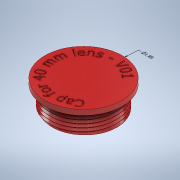
# Autodesk Inventor part: CapForSvBonyPlosse-40mm
Saved by Autodesk Inventor 2021.1 (Build 251245010, 245A)
## iProperties
Created: 2020-10-08
Part Number: CapForSvBonyPlosse-40mm
Material: PC/ABS Plastic
Document SubType Name: Modeling
Designer: robst
Density: 0.357273 g/cm^3
Appearance: Red
Author: robst
Autodesk Inventor part; units mm, degrees
ref_plane "YZ Plane" through (0, 0, 0) normal (1, 0, 0) x (0, 1, 0)
ref_plane "XZ Plane" through (0, 0, 0) normal (0, 1, 0) x (-1, 0, 0)
ref_plane "XY Plane" through (0, 0, 0) normal (0, 0, 1) x (1, 0, 0)
sketch "Sketch7" plane through (0, 0, 0) normal (0, 0, 1) x (1, 0, 0)
  line L0 (0, 0) -> (20.3518, 0)
  line L1 (20.3518, 0) -> (20.3517, 12.7)
  line L2 (20.3517, 12.7) -> (23.5267, 12.7)
  line L3 (23.5267, 12.7) -> (23.5267, 15.875)
  line L4 (23.5267, 15.875) -> (0, 15.875)
  line L5 (20.3518, 0) -> (17.1768, 0)
  line L6 (17.1768, 0) -> (17.1768, 12.7)
  line L7 (17.1768, 12.7) -> (0, 12.7)
  line L8 (0, 15.875) -> (0, 12.7)
  line L9 (0, -10.4241) -> (0, 20.2582) projected
  dimension "d71" = 3.175
  dimension "d72" = 12.7
  dimension "d73" = 20.3517
  dimension "d77" = 3.175
  dimension "d78" = 3.175
  constraints: 18 end point, 5 perpendicular, 2 vertical, 1 horizontal, 1 point on line
  measures "d71" distance between parallel lines of L4 L2
  measures "d72" distance from line of L2 L0.start
  measures "d73" distance of L0.start L0.end
  measures "d77" distance of L2.end L1.end
  measures "d78" distance between parallel lines of L1 L6
revolve "Revolution3" add sketch "Sketch7" angle 360 about axis through (0, -10, 0) along (0, 1, 0) contours L6 L7 L8 L4 L3 L2 L1 L0
sketch "Sketch10" plane through (0, 0, 0) normal (0, 0, 1) x (1, 0, 0)
  line L0 (20.3517, 12.7) -> (20.3517, 0) projected
  line L1 (20.3517, -2.1167) -> (20.3517, -4.1301)
  line L2 (20.3517, -4.1301) -> (18.9433, -3.317)
  line L3 (18.9433, -2.9298) -> (20.3517, -2.1167)
  line L4 (-20.3518, 0) -> (20.3517, 0) projected
  arc A0 (18.9433, -2.9298) -> (18.9433, -3.317) centre (19.0551, -3.1234) ccw
  line L5 (0, -7.921) -> (0, 19.841) projected
  point P0 (0, 0)
  dimension "d100" = 60
  dimension "d101" = 2.1167
  dimension "d102" = 0.2235
  dimension "d103" = 18.8316
  constraints: 6 end point, 2 point on circle, 2 tangent, 1 centre point, 1 collinear, 1 equal length, 1 vertical
  measures "d100" angle of L3 L2
  measures "d101" distance from line of L1.start L4
  measures "d102" radius of A0
  measures "d103" distance edge to line of A0 L5
coil "Coil6" sketch "Sketch10" operation cut axis through (0, -10, 0) along (0, 1, 0) pitch 2.1167 turns 8 hand right
sketch "Sketch11" plane through (0, 15.875, 0) normal (0, 1, 0) x (1, 0, 0)
  circle A0 centre (0, 0) radius 19.05 construction
  spline S0 degree 2 poles (10.2758, -12.8128) (10.6535, -12.4944) (11.5074, -12.2107) (11.9552, -12.2693) knots 0 0 0 1 2 2 2
  spline S1 degree 2 poles (11.9552, -12.2693) (12.4004, -12.3248) (13.2921, -12.8653) (13.7061, -13.3563) knots 0 0 0 1 2 2 2
  spline S2 degree 2 poles (13.7061, -13.3563) (14.1173, -13.8442) (14.4789, -14.7777) (14.4684, -15.2443) knots 0 0 0 1 2 2 2
  spline S3 degree 2 poles (14.4684, -15.2443) (14.4557, -15.7018) (14.0507, -16.5116) (13.6573, -16.8433) knots 0 0 0 1 2 2 2
  spline S4 degree 2 poles (13.6573, -16.8433) (13.4621, -17.0078) (13.0713, -17.2404) (12.8893, -17.3184) knots 0 0 0 1 2 2 2
  spline S5 degree 2 poles (12.8893, -17.3184) (12.729, -17.3836) (12.3695, -17.4873) (12.1821, -17.5269) knots 0 0 0 1 2 2 2
  line L0 (12.1821, -17.5269) -> (11.6568, -16.9037)
  line L1 (11.6568, -16.9037) -> (11.6977, -16.8692)
  spline S6 degree 2 poles (11.6977, -16.8692) (11.82, -16.8737) (12.1826, -16.8696) (12.4085, -16.8245) knots 0 0 0 1 2 2 2
  spline S7 degree 2 poles (12.4085, -16.8245) (12.6254, -16.7817) (13.0623, -16.591) (13.289, -16.4) knots 0 0 0 1 2 2 2
  spline S8 degree 2 poles (13.289, -16.4) (13.5376, -16.1904) (13.809, -15.6117) (13.8113, -15.2759) knots 0 0 0 1 2 2 2
  spline S9 degree 2 poles (13.8113, -15.2759) (13.8078, -14.9396) (13.4836, -14.1846) (13.1678, -13.81) knots 0 0 0 1 2 2 2
  spline S10 degree 2 poles (13.1678, -13.81) (12.8309, -13.4103) (12.1533, -12.9961) (11.8193, -12.9384) knots 0 0 0 1 2 2 2
  spline S11 degree 2 poles (11.8193, -12.9384) (11.4938, -12.8844) (10.8918, -13.0581) (10.6463, -13.265) knots 0 0 0 1 2 2 2
  spline S12 degree 2 poles (10.6463, -13.265) (10.4228, -13.4534) (10.1348, -13.8846) (10.0559, -14.0912) knots 0 0 0 1 2 2 2
  spline S13 degree 2 poles (10.0559, -14.0912) (9.9832, -14.2924) (9.9156, -14.6401) (9.9062, -14.7504) knots 0 0 0 1 2 2 2
  line L2 (9.9062, -14.7504) -> (9.8684, -14.7822)
  line L3 (9.8684, -14.7822) -> (9.3484, -14.1653)
  spline S14 degree 2 poles (9.3484, -14.1653) (9.427, -13.9967) (9.5608, -13.6955) (9.6789, -13.5098) knots 0 0 0 1 2 2 2
  spline S15 degree 2 poles (9.6789, -13.5098) (9.8011, -13.3099) (10.0429, -13.0091) (10.2758, -12.8128) knots 0 0 0 1 2 2 2
  spline S16 degree 2 poles (6.8845, -15.4673) (6.9287, -15.3808) (7.0724, -15.0789) (7.1552, -14.9685) knots 0 0 0 1 2 2 2
  spline S17 degree 2 poles (7.1552, -14.9685) (7.2657, -14.812) (7.507, -14.5856) (7.7647, -14.4568) knots 0 0 0 1 2 2 2
  spline S18 degree 2 poles (7.7647, -14.4568) (7.9747, -14.3519) (8.4331, -14.3208) (8.6485, -14.3926) knots 0 0 0 1 2 2 2
  spline S19 degree 2 poles (8.6485, -14.3926) (8.8546, -14.4645) (9.2265, -14.7941) (9.3405, -15.0224) knots 0 0 0 1 2 2 2
  spline S20 degree 2 poles (9.3405, -15.0224) (9.5172, -15.3759) (9.4692, -16.0258) (9.2169, -16.3314) knots 0 0 0 1 2 2 2
  spline S21 degree 2 poles (9.2169, -16.3314) (8.9959, -16.6075) (8.2649, -17.097) (7.8248, -17.3491) knots 0 0 0 1 2 2 2
  line L4 (7.8248, -17.3491) -> (7.88, -17.4596)
  spline S22 degree 2 poles (7.88, -17.4596) (7.9794, -17.6585) (8.2242, -17.8445) (8.3696, -17.8592) knots 0 0 0 1 2 2 2
  spline S23 degree 2 poles (8.3696, -17.8592) (8.5151, -17.874) (8.8538, -17.7599) (9.0232, -17.6753) knots 0 0 0 1 2 2 2
  spline S24 degree 2 poles (9.0232, -17.6753) (9.2221, -17.5759) (9.7009, -17.1894) (9.9126, -16.9409) knots 0 0 0 1 2 2 2
  line L5 (9.9126, -16.9409) -> (9.9458, -16.9244)
  line L6 (9.9458, -16.9244) -> (10.2384, -17.5099)
  spline S25 degree 2 poles (10.2384, -17.5099) (10.1021, -17.6332) (9.5644, -18.0399) (9.2735, -18.1853) knots 0 0 0 1 2 2 2
  spline S26 degree 2 poles (9.2735, -18.1853) (8.92, -18.362) (8.3824, -18.4925) (8.1191, -18.4446) knots 0 0 0 1 2 2 2
  spline S27 degree 2 poles (8.1191, -18.4446) (7.8614, -18.3985) (7.4546, -18.0449) (7.2945, -17.7246) knots 0 0 0 1 2 2 2
  line L7 (7.2945, -17.7246) -> (6.1297, -15.3935)
  line L8 (6.1297, -15.3935) -> (6.7041, -15.1065)
  line L9 (6.7041, -15.1065) -> (6.8845, -15.4673)
  line L10 (7.1237, -15.9461) -> (7.5966, -16.8925)
  spline S28 degree 2 poles (7.5966, -16.8925) (7.7936, -16.771) (8.3847, -16.3974) (8.5504, -16.241) knots 0 0 0 1 2 2 2
  spline S29 degree 2 poles (8.5504, -16.241) (8.7438, -16.0569) (8.8967, -15.617) (8.7679, -15.3592) knots 0 0 0 1 2 2 2
  spline S30 degree 2 poles (8.7679, -15.3592) (8.6207, -15.0646) (8.1402, -14.9319) (7.8235, -15.0902) knots 0 0 0 1 2 2 2
  spline S31 degree 2 poles (7.8235, -15.0902) (7.5547, -15.2245) (7.2287, -15.6773) (7.1237, -15.9461) knots 0 0 0 1 2 2 2
  spline S32 degree 2 poles (2.6555, -18.4089) (2.4319, -17.4804) (3.0523, -16.1708) (3.7286, -16.0079) knots 0 0 0 1 2 2 2
  spline S33 degree 2 poles (3.7286, -16.0079) (4.0048, -15.9413) (4.4599, -15.9672) (4.7118, -16.0463) knots 0 0 0 1 2 2 2
  line L11 (4.7118, -16.0463) -> (4.3378, -14.4934)
  line L12 (4.3378, -14.4934) -> (4.9621, -14.343)
  line L13 (4.9621, -14.343) -> (6.1835, -19.4139)
  line L14 (6.1835, -19.4139) -> (5.5592, -19.5642)
  line L15 (5.5592, -19.5642) -> (5.4657, -19.176)
  spline S34 degree 2 poles (5.4657, -19.176) (5.2846, -19.4441) (4.7838, -19.8611) (4.4516, -19.9411) knots 0 0 0 1 2 2 2
  spline S35 degree 2 poles (4.4516, -19.9411) (3.8152, -20.0944) (2.8599, -19.2574) (2.6555, -18.4089) knots 0 0 0 1 2 2 2
  spline S36 degree 2 poles (3.2826, -18.1817) (3.4358, -18.8181) (4.0088, -19.4211) (4.461, -19.3121) knots 0 0 0 1 2 2 2
  spline S37 degree 2 poles (4.461, -19.3121) (4.7252, -19.2485) (5.1646, -18.8929) (5.3403, -18.6557) knots 0 0 0 1 2 2 2
  line L16 (5.3403, -18.6557) -> (4.8333, -16.5506)
  spline S38 degree 2 poles (4.8333, -16.5506) (4.5612, -16.4933) (4.1918, -16.4891) (3.9677, -16.5431) knots 0 0 0 1 2 2 2
  spline S39 degree 2 poles (3.9677, -16.5431) (3.4834, -16.6597) (3.1187, -17.5013) (3.2826, -18.1817) knots 0 0 0 1 2 2 2
  line L17 (-3.0523, -21.0173) -> (-3.0195, -21.0201)
  spline S40 degree 2 poles (-3.0195, -21.0201) (-2.9361, -21.0601) (-2.6209, -21.1444) (-2.4937, -21.1551) knots 0 0 0 1 2 2 2
  spline S41 degree 2 poles (-2.4937, -21.1551) (-2.0917, -21.1888) (-1.7168, -20.8567) (-1.6769, -20.3808) knots 0 0 0 1 2 2 2
  line L18 (-1.6769, -20.3808) -> (-1.6662, -20.2537)
  line L19 (-1.6662, -20.2537) -> (-2.7246, -20.1649)
  line L20 (-2.7246, -20.1649) -> (-2.6802, -19.6357)
  line L21 (-2.6802, -19.6357) -> (-1.6424, -19.7227)
  line L22 (-1.6424, -19.7227) -> (-1.368, -16.4532)
  line L23 (-1.368, -16.4532) -> (-0.7281, -16.5069)
  line L24 (-0.7281, -16.5069) -> (-1.0024, -19.7764)
  line L25 (-1.0024, -19.7764) -> (-0.5717, -19.8126)
  line L26 (-0.5717, -19.8126) -> (-0.6161, -20.3418)
  line L27 (-0.6161, -20.3418) -> (-1.0468, -20.3056)
  line L28 (-1.0468, -20.3056) -> (-1.0575, -20.4328)
  spline S42 degree 2 poles (-1.0575, -20.4328) (-1.1146, -21.1138) (-1.835, -21.7722) (-2.4503, -21.7205) knots 0 0 0 1 2 2 2
  spline S43 degree 2 poles (-2.4503, -21.7205) (-2.6267, -21.7057) (-2.9641, -21.6402) (-3.1015, -21.6039) knots 0 0 0 1 2 2 2
  line L29 (-3.1015, -21.6039) -> (-3.0523, -21.0173)
  spline S44 degree 2 poles (-6.5478, -17.2966) (-6.2911, -16.3682) (-5.1186, -15.6032) (-4.3727, -15.8094) knots 0 0 0 1 2 2 2
  spline S45 degree 2 poles (-4.3727, -15.8094) (-3.6069, -16.0211) (-3.0185, -17.3071) (-3.2664, -18.2038) knots 0 0 0 1 2 2 2
  spline S46 degree 2 poles (-3.2664, -18.2038) (-3.5209, -19.1243) (-4.7074, -19.894) (-5.4455, -19.69) knots 0 0 0 1 2 2 2
  spline S47 degree 2 poles (-5.4455, -19.69) (-6.1914, -19.4837) (-6.8034, -18.2212) (-6.5478, -17.2966) knots 0 0 0 1 2 2 2
  spline S48 degree 2 poles (-5.909, -17.4733) (-6.1064, -18.1875) (-5.7786, -19.0255) (-5.2985, -19.1583) knots 0 0 0 1 2 2 2
  spline S49 degree 2 poles (-5.2985, -19.1583) (-4.8184, -19.291) (-4.1027, -18.7414) (-3.9052, -18.0272) knots 0 0 0 1 2 2 2
  spline S50 degree 2 poles (-3.9052, -18.0272) (-3.7132, -17.3328) (-4.0396, -16.4738) (-4.5197, -16.3411) knots 0 0 0 1 2 2 2
  spline S51 degree 2 poles (-4.5197, -16.3411) (-4.9958, -16.2095) (-5.7137, -16.767) (-5.909, -17.4733) knots 0 0 0 1 2 2 2
  line L30 (-9.8192, -17.0471) -> (-9.7897, -17.0617)
  spline S52 degree 2 poles (-9.7897, -17.0617) (-9.7325, -17.1131) (-9.5923, -17.1918) (-9.4927, -17.2411) knots 0 0 0 1 2 2 2
  spline S53 degree 2 poles (-9.4927, -17.2411) (-9.2603, -17.3563) (-8.7024, -17.3802) (-8.3971, -17.2834) knots 0 0 0 1 2 2 2
  line L31 (-8.3971, -17.2834) -> (-7.1959, -14.8601)
  line L32 (-7.1959, -14.8601) -> (-6.6205, -15.1453)
  line L33 (-6.6205, -15.1453) -> (-8.3136, -18.5608)
  line L34 (-8.3136, -18.5608) -> (-8.8889, -18.2756)
  line L35 (-8.8889, -18.2756) -> (-8.6366, -17.7666)
  spline S54 degree 2 poles (-8.6366, -17.7666) (-9.0891, -17.8915) (-9.6709, -17.888) (-9.8922, -17.7783) knots 0 0 0 1 2 2 2
  spline S55 degree 2 poles (-9.8922, -17.7783) (-9.9807, -17.7344) (-10.0656, -17.6831) (-10.1154, -17.6446) knots 0 0 0 1 2 2 2
  line L36 (-10.1154, -17.6446) -> (-9.8192, -17.0471)
  line L37 (-14.1089, -11.7135) -> (-13.68, -12.1405)
  line L38 (-13.68, -12.1405) -> (-12.4485, -10.9036)
  line L39 (-12.4485, -10.9036) -> (-11.9846, -11.3654)
  line L40 (-11.9846, -11.3654) -> (-13.2162, -12.6023)
  line L41 (-13.2162, -12.6023) -> (-11.6263, -14.1854)
  line L42 (-11.6263, -14.1854) -> (-12.1317, -14.693)
  line L43 (-12.1317, -14.693) -> (-15.5894, -14.9449)
  line L44 (-15.5894, -14.9449) -> (-16.0328, -14.5034)
  line L45 (-16.0328, -14.5034) -> (-14.0664, -12.5285)
  line L46 (-14.0664, -12.5285) -> (-14.4952, -12.1015)
  line L47 (-14.4952, -12.1015) -> (-14.1089, -11.7135)
  line L48 (-13.6025, -12.9903) -> (-15.0026, -14.3964)
  line L49 (-15.0026, -14.3964) -> (-12.3919, -14.1958)
  line L50 (-12.3919, -14.1958) -> (-13.6025, -12.9903)
  spline S56 degree 2 poles (-17.0242, -8.7019) (-15.8646, -7.9786) (-14.3578, -7.9752) (-13.9199, -8.6772) knots 0 0 0 1 2 2 2
  spline S57 degree 2 poles (-13.9199, -8.6772) (-13.4754, -9.3898) (-14.1666, -10.7476) (-15.3018, -11.4556) knots 0 0 0 1 2 2 2
  spline S58 degree 2 poles (-15.3018, -11.4556) (-16.4684, -12.1833) (-17.9682, -12.1823) (-18.4083, -11.4768) knots 0 0 0 1 2 2 2
  spline S59 degree 2 poles (-18.4083, -11.4768) (-18.8506, -10.7677) (-18.149, -9.4034) (-17.0242, -8.7019) knots 0 0 0 1 2 2 2
  spline S60 degree 2 poles (-15.249, -8.6232) (-15.5144, -8.6723) (-16.2146, -9.012) (-16.6582, -9.2887) knots 0 0 0 1 2 2 2
  spline S61 degree 2 poles (-16.6582, -9.2887) (-17.1018, -9.5654) (-17.7114, -10.0426) (-17.877, -10.2672) knots 0 0 0 1 2 2 2
  spline S62 degree 2 poles (-17.877, -10.2672) (-18.0426, -10.4918) (-18.0801, -10.9373) (-17.9298, -11.1783) knots 0 0 0 1 2 2 2
  spline S63 degree 2 poles (-17.9298, -11.1783) (-17.7795, -11.4193) (-17.3585, -11.5886) (-17.0748, -11.5378) knots 0 0 0 1 2 2 2
  spline S64 degree 2 poles (-17.0748, -11.5378) (-16.8003, -11.4879) (-16.0905, -11.1324) (-15.6678, -10.8688) knots 0 0 0 1 2 2 2
  spline S65 degree 2 poles (-15.6678, -10.8688) (-15.2137, -10.5856) (-14.6408, -10.1506) (-14.4599, -9.9117) knots 0 0 0 1 2 2 2
  spline S66 degree 2 poles (-14.4599, -9.9117) (-14.2887, -9.6884) (-14.2415, -9.2272) (-14.3984, -8.9757) knots 0 0 0 1 2 2 2
  spline S67 degree 2 poles (-14.3984, -8.9757) (-14.5466, -8.7382) (-14.9675, -8.5689) (-15.249, -8.6232) knots 0 0 0 1 2 2 2
  line L51 (-16.6094, -0.3836) -> (-18.7959, -0.6805)
  spline S68 degree 2 poles (-18.7959, -0.6805) (-19.057, -0.716) (-19.4961, -0.8171) (-19.6096, -0.899) knots 0 0 0 1 2 2 2
  spline S69 degree 2 poles (-19.6096, -0.899) (-19.7353, -0.9825) (-19.8321, -1.2491) (-19.8027, -1.4653) knots 0 0 0 1 2 2 2
  spline S70 degree 2 poles (-19.8027, -1.4653) (-19.7761, -1.6611) (-19.4745, -2.0772) (-19.214, -2.2827) knots 0 0 0 1 2 2 2
  spline S71 degree 2 poles (-19.214, -2.2827) (-19.1574, -2.2709) (-18.9994, -2.2411) (-18.8934, -2.2267) knots 0 0 0 1 2 2 2
  line L52 (-18.8934, -2.2267) -> (-16.405, -1.8889)
  line L53 (-16.405, -1.8889) -> (-16.3186, -2.5252)
  line L54 (-16.3186, -2.5252) -> (-18.5051, -2.8221)
  spline S72 degree 2 poles (-18.5051, -2.8221) (-18.7662, -2.8576) (-19.2053, -2.9587) (-19.3188, -3.0406) knots 0 0 0 1 2 2 2
  spline S73 degree 2 poles (-19.3188, -3.0406) (-19.4445, -3.1242) (-19.5413, -3.3907) (-19.5119, -3.6069) knots 0 0 0 1 2 2 2
  spline S74 degree 2 poles (-19.5119, -3.6069) (-19.4842, -3.8109) (-19.1658, -4.2288) (-18.9371, -4.4138) knots 0 0 0 1 2 2 2
  line L55 (-18.9371, -4.4138) -> (-16.1142, -4.0305)
  line L56 (-16.1142, -4.0305) -> (-16.0278, -4.6669)
  line L57 (-16.0278, -4.6669) -> (-19.8052, -5.1797)
  line L58 (-19.8052, -5.1797) -> (-19.8916, -4.5434)
  line L59 (-19.8916, -4.5434) -> (-19.4756, -4.4869)
  spline S75 degree 2 poles (-19.4756, -4.4869) (-19.7582, -4.2718) (-20.0979, -3.8194) (-20.1378, -3.5257) knots 0 0 0 1 2 2 2
  spline S76 degree 2 poles (-20.1378, -3.5257) (-20.1832, -3.1912) (-19.9476, -2.6316) (-19.6192, -2.4499) knots 0 0 0 1 2 2 2
  spline S77 degree 2 poles (-19.6192, -2.4499) (-19.9808, -2.2041) (-20.3854, -1.7023) (-20.4286, -1.3841) knots 0 0 0 1 2 2 2
  spline S78 degree 2 poles (-20.4286, -1.3841) (-20.4618, -1.1394) (-20.3652, -0.7191) (-20.2138, -0.549) knots 0 0 0 1 2 2 2
  spline S79 degree 2 poles (-20.2138, -0.549) (-20.063, -0.3748) (-19.5717, -0.1377) (-19.1842, -0.0851) knots 0 0 0 1 2 2 2
  line L60 (-19.1842, -0.0851) -> (-16.6958, 0.2527)
  line L61 (-16.6958, 0.2527) -> (-16.6094, -0.3836)
  line L62 (-15.7252, 5.3609) -> (-17.8801, 5.8353)
  spline S80 degree 2 poles (-17.8801, 5.8353) (-18.1374, 5.8919) (-18.5845, 5.9482) (-18.7193, 5.9104) knots 0 0 0 1 2 2 2
  spline S81 degree 2 poles (-18.7193, 5.9104) (-18.8661, 5.8753) (-19.0487, 5.6584) (-19.0956, 5.4453) knots 0 0 0 1 2 2 2
  spline S82 degree 2 poles (-19.0956, 5.4453) (-19.1381, 5.2523) (-18.9983, 4.7579) (-18.8245, 4.4751) knots 0 0 0 1 2 2 2
  spline S83 degree 2 poles (-18.8245, 4.4751) (-18.7673, 4.4668) (-18.6087, 4.4403) (-18.5042, 4.4173) knots 0 0 0 1 2 2 2
  line L63 (-18.5042, 4.4173) -> (-16.0518, 3.8774)
  line L64 (-16.0518, 3.8774) -> (-16.1898, 3.2502)
  line L65 (-16.1898, 3.2502) -> (-18.3448, 3.7246)
  spline S84 degree 2 poles (-18.3448, 3.7246) (-18.6021, 3.7812) (-19.0492, 3.8375) (-19.1839, 3.7997) knots 0 0 0 1 2 2 2
  spline S85 degree 2 poles (-19.1839, 3.7997) (-19.3308, 3.7646) (-19.5134, 3.5477) (-19.5603, 3.3346) knots 0 0 0 1 2 2 2
  spline S86 degree 2 poles (-19.5603, 3.3346) (-19.6046, 3.1336) (-19.4495, 2.6316) (-19.2986, 2.3791) knots 0 0 0 1 2 2 2
  line L66 (-19.2986, 2.3791) -> (-16.5164, 1.7666)
  line L67 (-16.5164, 1.7666) -> (-16.6545, 1.1394)
  line L68 (-16.6545, 1.1394) -> (-20.3774, 1.9591)
  line L69 (-20.3774, 1.9591) -> (-20.2393, 2.5862)
  line L70 (-20.2393, 2.5862) -> (-19.8293, 2.496)
  spline S87 degree 2 poles (-19.8293, 2.496) (-20.0205, 2.7952) (-20.1837, 3.3369) (-20.1199, 3.6264) knots 0 0 0 1 2 2 2
  spline S88 degree 2 poles (-20.1199, 3.6264) (-20.0474, 3.9561) (-19.6334, 4.4003) (-19.2625, 4.4577) knots 0 0 0 1 2 2 2
  spline S89 degree 2 poles (-19.2625, 4.4577) (-19.5172, 4.8131) (-19.7243, 5.4235) (-19.6553, 5.7371) knots 0 0 0 1 2 2 2
  spline S90 degree 2 poles (-19.6553, 5.7371) (-19.6022, 5.9784) (-19.3667, 6.3396) (-19.1659, 6.4472) knots 0 0 0 1 2 2 2
  spline S91 degree 2 poles (-19.1659, 6.4472) (-18.9643, 6.5588) (-18.4215, 6.6121) (-18.0395, 6.528) knots 0 0 0 1 2 2 2
  line L71 (-18.0395, 6.528) -> (-15.5871, 5.9881)
  line L72 (-15.5871, 5.9881) -> (-15.7252, 5.3609)
  line L73 (-13.7006, 9.2183) -> (-14.0487, 8.6786)
  line L74 (-14.0487, 8.6786) -> (-18.5081, 11.5546)
  line L75 (-18.5081, 11.5546) -> (-18.16, 12.0943)
  line L76 (-18.16, 12.0943) -> (-13.7006, 9.2183)
  spline S92 degree 2 poles (-12.0277, 11.1869) (-12.6385, 10.5071) (-14.0724, 10.4451) (-14.7767, 11.0779) knots 0 0 0 1 2 2 2
  spline S93 degree 2 poles (-14.7767, 11.0779) (-15.4687, 11.6998) (-15.6372, 13.1629) (-15.1117, 13.7478) knots 0 0 0 1 2 2 2
  spline S94 degree 2 poles (-15.1117, 13.7478) (-14.875, 14.0111) (-14.356, 14.2808) (-14.0589, 14.285) knots 0 0 0 1 2 2 2
  spline S95 degree 2 poles (-14.0589, 14.285) (-13.759, 14.2923) (-13.1447, 14.0336) (-12.8048, 13.7282) knots 0 0 0 1 2 2 2
  line L77 (-12.8048, 13.7282) -> (-12.5445, 13.4943)
  line L78 (-12.5445, 13.4943) -> (-14.3082, 11.5315)
  spline S96 degree 2 poles (-14.3082, 11.5315) (-13.8152, 11.0885) (-12.8459, 11.114) (-12.4497, 11.555) knots 0 0 0 1 2 2 2
  spline S97 degree 2 poles (-12.4497, 11.555) (-12.3093, 11.7111) (-12.1074, 12.0776) (-12.0524, 12.2496) knots 0 0 0 1 2 2 2
  spline S98 degree 2 poles (-12.0524, 12.2496) (-11.9981, 12.4332) (-11.9457, 12.7071) (-11.9424, 12.8093) knots 0 0 0 1 2 2 2
  line L79 (-11.9424, 12.8093) -> (-11.9176, 12.8369)
  line L80 (-11.9176, 12.8369) -> (-11.3971, 12.3691)
  spline S99 degree 2 poles (-11.3971, 12.3691) (-11.4377, 12.2562) (-11.5653, 11.9171) (-11.6258, 11.7943) knots 0 0 0 1 2 2 2
  spline S100 degree 2 poles (-11.6258, 11.7943) (-11.7098, 11.6207) (-11.8736, 11.3584) (-12.0277, 11.1869) knots 0 0 0 1 2 2 2
  spline S101 degree 2 poles (-13.3271, 13.3563) (-13.5255, 13.5235) (-13.8788, 13.697) (-14.0425, 13.7058) knots 0 0 0 1 2 2 2
  spline S102 degree 2 poles (-14.0425, 13.7058) (-14.224, 13.7194) (-14.5711, 13.5609) (-14.7445, 13.368) knots 0 0 0 1 2 2 2
  spline S103 degree 2 poles (-14.7445, 13.368) (-14.9151, 13.1782) (-15.0412, 12.8099) (-15.03, 12.6007) knots 0 0 0 1 2 2 2
  spline S104 degree 2 poles (-15.03, 12.6007) (-15.013, 12.3917) (-14.8395, 12.0366) (-14.6726, 11.8589) knots 0 0 0 1 2 2 2
  line L81 (-14.6726, 11.8589) -> (-13.3271, 13.3563)
  line L82 (-8.2268, 14.3938) -> (-8.753, 14.0257)
  line L83 (-8.753, 14.0257) -> (-9.9991, 15.8066)
  spline S105 degree 2 poles (-9.9991, 15.8066) (-10.1501, 16.0225) (-10.4502, 16.3652) (-10.5888, 16.4341) knots 0 0 0 1 2 2 2
  spline S106 degree 2 poles (-10.5888, 16.4341) (-10.7355, 16.5073) (-11.0451, 16.4615) (-11.2407, 16.3246) knots 0 0 0 1 2 2 2
  spline S107 degree 2 poles (-11.2407, 16.3246) (-11.4364, 16.1877) (-11.705, 15.6883) (-11.786, 15.3804) knots 0 0 0 1 2 2 2
  line L84 (-11.786, 15.3804) -> (-10.1529, 13.0463)
  line L85 (-10.1529, 13.0463) -> (-10.6791, 12.6781)
  line L86 (-10.6791, 12.6781) -> (-12.8644, 15.8016)
  line L87 (-12.8644, 15.8016) -> (-12.3382, 16.1697)
  line L88 (-12.3382, 16.1697) -> (-12.0951, 15.8223)
  spline S108 degree 2 poles (-12.0951, 15.8223) (-12.0077, 16.2) (-11.7081, 16.7412) (-11.4517, 16.9206) knots 0 0 0 1 2 2 2
  spline S109 degree 2 poles (-11.4517, 16.9206) (-10.993, 17.2415) (-10.0487, 16.9978) (-9.6452, 16.421) knots 0 0 0 1 2 2 2
  line L89 (-9.6452, 16.421) -> (-8.2268, 14.3938)
  spline S110 degree 2 poles (-6.4377, 15.1049) (-6.7905, 14.9562) (-7.4812, 14.8883) (-7.727, 14.9098) knots 0 0 0 1 2 2 2
  line L90 (-7.727, 14.9098) -> (-8.0069, 15.5736)
  line L91 (-8.0069, 15.5736) -> (-7.9765, 15.5864)
  spline S111 degree 2 poles (-7.9765, 15.5864) (-7.8751, 15.5577) (-7.6094, 15.4999) (-7.4052, 15.4922) knots 0 0 0 1 2 2 2
  spline S112 degree 2 poles (-7.4052, 15.4922) (-7.2268, 15.4825) (-6.8179, 15.5299) (-6.6244, 15.6114) knots 0 0 0 1 2 2 2
  spline S113 degree 2 poles (-6.6244, 15.6114) (-6.4841, 15.6706) (-6.1888, 15.871) (-6.1354, 15.9561) knots 0 0 0 1 2 2 2
  spline S114 degree 2 poles (-6.1354, 15.9561) (-6.0557, 16.0746) (-6.0259, 16.2793) (-6.0963, 16.4462) knots 0 0 0 1 2 2 2
  spline S115 degree 2 poles (-6.0963, 16.4462) (-6.1842, 16.6548) (-6.503, 16.7751) (-6.8255, 16.724) knots 0 0 0 1 2 2 2
  spline S116 degree 2 poles (-6.8255, 16.724) (-6.9504, 16.7026) (-7.3466, 16.6249) (-7.5197, 16.6011) knots 0 0 0 1 2 2 2
  spline S117 degree 2 poles (-7.5197, 16.6011) (-7.9714, 16.5491) (-8.5403, 16.8811) (-8.6858, 17.2263) knots 0 0 0 1 2 2 2
  spline S118 degree 2 poles (-8.6858, 17.2263) (-8.8873, 17.7043) (-8.4215, 18.6021) (-7.8297, 18.8516) knots 0 0 0 1 2 2 2
  spline S119 degree 2 poles (-7.8297, 18.8516) (-7.5376, 18.9748) (-6.8851, 19.0801) (-6.6377, 19.0549) knots 0 0 0 1 2 2 2
  line L92 (-6.6377, 19.0549) -> (-6.3706, 18.4214)
  line L93 (-6.3706, 18.4214) -> (-6.4009, 18.4086)
  spline S120 degree 2 poles (-6.4009, 18.4086) (-6.7053, 18.4947) (-7.3471, 18.4698) (-7.6316, 18.3499) knots 0 0 0 1 2 2 2
  spline S121 degree 2 poles (-7.6316, 18.3499) (-7.9237, 18.2267) (-8.2218, 17.8106) (-8.1178, 17.5641) knots 0 0 0 1 2 2 2
  spline S122 degree 2 poles (-8.1178, 17.5641) (-8.0235, 17.3403) (-7.6933, 17.2248) (-7.399, 17.2685) knots 0 0 0 1 2 2 2
  spline S123 degree 2 poles (-7.399, 17.2685) (-7.2557, 17.2887) (-6.9006, 17.358) (-6.7048, 17.3914) knots 0 0 0 1 2 2 2
  spline S124 degree 2 poles (-6.7048, 17.3914) (-6.2763, 17.4559) (-5.6914, 17.1708) (-5.5267, 16.7801) knots 0 0 0 1 2 2 2
  spline S125 degree 2 poles (-5.5267, 16.7801) (-5.4307, 16.5525) (-5.4395, 16.0753) (-5.5516, 15.8538) knots 0 0 0 1 2 2 2
  spline S126 degree 2 poles (-5.5516, 15.8538) (-5.6719, 15.6199) (-6.0773, 15.2568) (-6.4377, 15.1049) knots 0 0 0 1 2 2 2
  line L94 (-0.8125, 18.4315) -> (-2.7261, 18.2467)
  line L95 (-2.7261, 18.2467) -> (-2.7855, 18.8613)
  line L96 (-2.7855, 18.8613) -> (-0.8719, 19.0462)
  line L97 (-0.8719, 19.0462) -> (-0.8125, 18.4315)
  line L98 (7.1505, 20.478) -> (4.245, 15.9585)
  line L99 (4.245, 15.9585) -> (3.5372, 16.1314)
  line L100 (3.5372, 16.1314) -> (3.0435, 21.4815)
  line L101 (3.0435, 21.4815) -> (3.7473, 21.3096)
  line L102 (3.7473, 21.3096) -> (4.1133, 16.8763)
  line L103 (4.1133, 16.8763) -> (6.4826, 20.6411)
  line L104 (6.4826, 20.6411) -> (7.1505, 20.478)
  spline S127 degree 2 poles (10.2707, 16.1264) (9.6372, 14.9153) (8.3397, 14.1491) (7.6065, 14.5327) knots 0 0 0 1 2 2 2
  spline S128 degree 2 poles (7.6065, 14.5327) (6.8624, 14.9219) (6.7705, 16.4427) (7.3907, 17.6282) knots 0 0 0 1 2 2 2
  spline S129 degree 2 poles (7.3907, 17.6282) (8.028, 18.8466) (9.3216, 19.6055) (10.0585, 19.22) knots 0 0 0 1 2 2 2
  spline S130 degree 2 poles (10.0585, 19.22) (10.799, 18.8327) (10.8851, 17.301) (10.2707, 16.1264) knots 0 0 0 1 2 2 2
  spline S131 degree 2 poles (8.7799, 15.1593) (8.9838, 15.3361) (9.4155, 15.9837) (9.6578, 16.4469) knots 0 0 0 1 2 2 2
  spline S132 degree 2 poles (9.6578, 16.4469) (9.9002, 16.9102) (10.184, 17.6305) (10.2131, 17.908) knots 0 0 0 1 2 2 2
  spline S133 degree 2 poles (10.2131, 17.908) (10.2421, 18.1855) (10.0487, 18.5886) (9.797, 18.7203) knots 0 0 0 1 2 2 2
  spline S134 degree 2 poles (9.797, 18.7203) (9.5453, 18.852) (9.0967, 18.7847) (8.8778, 18.5972) knots 0 0 0 1 2 2 2
  spline S135 degree 2 poles (8.8778, 18.5972) (8.6664, 18.4151) (8.2344, 17.749) (8.0035, 17.3077) knots 0 0 0 1 2 2 2
  spline S136 degree 2 poles (8.0035, 17.3077) (7.7554, 16.8335) (7.4818, 16.1682) (7.4469, 15.8706) knots 0 0 0 1 2 2 2
  spline S137 degree 2 poles (7.4469, 15.8706) (7.4123, 15.5913) (7.6053, 15.1698) (7.8679, 15.0324) knots 0 0 0 1 2 2 2
  spline S138 degree 2 poles (7.8679, 15.0324) (8.116, 14.9026) (8.5647, 14.9699) (8.7799, 15.1593) knots 0 0 0 1 2 2 2
  line L105 (11.8008, 11.6243) -> (9.9243, 13.2431)
  line L106 (9.9243, 13.2431) -> (10.2631, 13.6358)
  line L107 (10.2631, 13.6358) -> (10.9613, 13.0335)
  line L108 (10.9613, 13.0335) -> (13.1852, 15.6113)
  line L109 (13.1852, 15.6113) -> (12.487, 16.2136)
  line L110 (12.487, 16.2136) -> (12.7909, 16.5659)
  spline S139 degree 2 poles (12.7909, 16.5659) (13.1867, 16.2243) (13.7544, 16.1261) (14.0482, 16.4163) knots 0 0 0 1 2 2 2
  line L111 (14.0482, 16.4163) -> (14.4472, 16.0721)
  line L112 (14.4472, 16.0721) -> (11.4569, 12.6059)
  line L113 (11.4569, 12.6059) -> (12.1396, 12.017)
  line L114 (12.1396, 12.017) -> (11.8008, 11.6243)
  dimension "d112" = 38.1
  constraints: 1 centre point, 1 coincident, 1 other
  measures "d112" diameter of A0
extrude "Extrusion1" cut sketch "Sketch11" against normal blind 1.27
equation "\"d71\" = wallThickness"
equation "\"d72\" = caseHeightAboveLens"
equation "\"d73\" = a1MajorRadiusAvg"
equation "\"d77\" = wallThickness"
equation "\"d78\" = wallThickness"
equation "\"d101\" = pitch"
equation "\"d102\" = a1RootRadiusAvg"
equation "\"d103\" = a1MinorRadiusAvg"
equation "\"d104\" = pitch"
equation "\"baseDiameter\" = 31.75"
equation "\"baseRadius\" = 0.5 * baseDiameter"
equation "\"baseHeight\" = 25.4"
equation "\"middleDiameter\" = 34.29"
equation "\"middleRadius\" = 0.5 * middleDiameter"
equation "\"middleTopDiameter\" = 34.798"
equation "\"middleTopRadius\" = 0.5 * middleTopDiameter"
equation "\"middleHeight\" = 18.542"
equation "\"middleTopHeight\" = 30.734"
equation "\"topBaseDiameter\" = 34.798"
equation "\"topHeightDiameter\" = 40.894"
equation "\"topBaseRadius\" = 0.5 * topBaseDiameter"
equation "\"topHeightRadius\" = 0.5 * topHeightDiameter"
equation "\"topHeight\" = 7.62"
equation "\"d9\" = caseBottomThickness"
equation "\"wallThickness\" = 3.175"
equation "\"caseBottomThickness\" = 4.7625"
equation "\"caseHeightAboveLens\" = 12.7"
equation "\"baseWallThickness\" = 2.032"
equation "\"baseInteriorHeight\" = 15.24"
equation "\"interiorDiameter\" = 41.275"
equation "\"outsideRadius\" = interiorRadius + wallThickness"
equation "\"outsideDiameter\" = 2 * outsideRadius"
equation "\"textRingDiameter\" = 0.75 * outsideDiameter"
equation "\"b2MajorDiameterMax\" = 41.275"
equation "\"b2MajorRadiusMax\" = 0.5 * b2MajorDiameterMax"
equation "\"a1MinorDiameterAvg\" = 37.66312"
equation "\"a1MinorRadiusAvg\" = 0.5 * a1MinorDiameterAvg"
equation "\"a1MajorDiameterAvg\" = 40.7035"
equation "\"a1MajorRadiusAvg\" = 0.5 * a1MajorDiameterAvg"
equation "\"a1RootRadiusAvg\" = 0.22352"
equation "\"pitch\" = 2.116667"
equation "\"interiorRadius\" = 20.6375"
body "Solid3"
